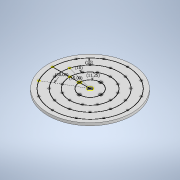
# Autodesk Inventor part: Part12
Saved by Autodesk Inventor 2021 (Build 250183000, 183)
## iProperties
Created: 2021-05-23
Part Number: Part12
Material: Generic
Document SubType Name: Modeling
Designer: dsdan
Density: 1 g/cm^3
Appearance: Default
Author: dsdan
Autodesk Inventor part; units mm, degrees
ref_plane "YZ Plane" through (0, 0, 0) normal (1, 0, 0) x (0, 1, 0)
ref_plane "XZ Plane" through (0, 0, 0) normal (0, 1, 0) x (-1, 0, 0)
ref_plane "XY Plane" through (0, 0, 0) normal (0, 0, 1) x (1, 0, 0)
sketch "Sketch1" plane through (0, 0, 0) normal (0, 1, 0) x (-1, 0, 0)
  circle A0 centre (0, 0) radius 49
  circle A1 centre (0, 0) radius 3
  circle A2 centre (0, 12.5) radius 2
  circle A3 centre (-12.5, 0) radius 2
  circle A4 centre (0, -12.5) radius 2
  circle A5 centre (12.5, 0) radius 2
  dimension "d0" = 98
  dimension "d1" = 6
  dimension "d6" = 12.5
  dimension "d9" = 360
  dimension "d11" = 4
  constraints: 6 centre point, 2 coincident, 1 vertical alignment, 9 other
  measures "d0" diameter of A0
  measures "d1" diameter of A1
  measures "d6" distance of A1.centre A2.centre
  measures "d11" diameter of A2
extrude "Extrusion1" add sketch "Sketch1" along normal blind 3
sketch "Sketch2" plane through (0, 3, 0) normal (0, 1, 0) x (1, 0, 0)
  circle A0 centre (-43.75, 0) radius 1.25
  circle A1 centre (0, 0) radius 49 construction
  circle A2 centre (-23.75, 0) radius 1.25
  circle A3 centre (-32.6, -8.7351) radius 1.25
  line L0 (0, 0) -> (-22.9407, -6.147) construction
  line L1 (0, 0) -> (-23.75, 0) construction
  arc A4 (-23.75, 0) -> (-22.9407, -6.147) centre (5.6453, 0.7432) ccw construction
  line L2 (-22.9407, -6.147) -> (-32.6, -8.7351) construction
  point P0 (-49, 0)
  dimension "d14" = 2.5
  dimension "d16" = 5.25
  dimension "d17" = 20
  dimension "d24" = 15
  dimension "d25" = 10
  constraints: 6 end point, 4 centre point, 4 horizontal alignment, 2 equal radius, 2 point on circle, 1 collinear, 1 equal length, 1 horizontal, 1 other
  measures "d14" diameter of A0
  measures "d16" distance of point (-49, 0) A0.centre
  measures "d17" distance of A0.centre L1.end
  measures "d24" angle of L1 L0
  measures "d25" distance of L0.end L2.end
extrude "Extrusion2" cut sketch "Sketch2" against normal through all
pattern_circular "Circular Pattern1" count 12 over 360 about axis through (0, 0, 0) along (0, 1, 0) of "Extrusion2"
sketch "Sketch3" plane through (0, 3, 0) normal (0, 1, 0) x (1, 0, 0)
  circle A0 centre (-43.75, 0) radius 1.25 projected
  line L0 (0, 0) -> (-43.75, 0)
  circle A1 centre (-37.8886, -21.875) radius 1.25 projected
  line L1 (-37.8886, -21.875) -> (0, 0) construction
  circle A2 centre (-32.6, 8.7351) radius 1.25 projected
  circle A3 centre (0, 0) radius 3 projected
  circle A4 centre (0, 0) radius 43.75
  circle A5 centre (-23.75, 0) radius 1.25 projected
  circle A6 centre (0, 0) radius 23.75
  circle A7 centre (0, 0) radius 33.75
  circle A8 centre (-12.5, 0) radius 2 projected
  circle A9 centre (0, 0) radius 12.5
  line L2 (0, 0) -> (-32.6, 8.7351) construction
  dimension "d28" = 10
  dimension "d29" = 10
  dimension "d30" = 11.25
  dimension "d23" = 30
  dimension "d31" = 15
  constraints: 6 end point, 4 coincident, 3 horizontal alignment, 1 horizontal, 9 other
  measures "d23" angle of L0 L1
  measures "d31" angle of L0 L2
equation "\"d25\" = 0.5 * d17"
body "Solid1"
